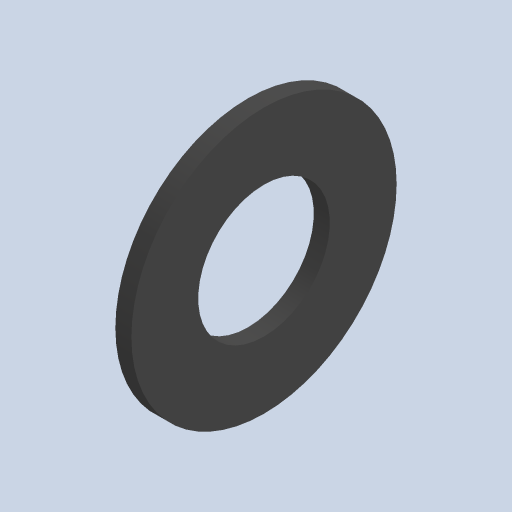
# Autodesk Inventor part: rubberWasher1
Saved by Autodesk Inventor 2023 (Build 270158030, 158C)
## iProperties
Created: 2023-01-21
Part Number: rubberWasher1
Material: Rubber
Document SubType Name: Modeling
Designer: kumpu
Density: 0.93 g/cm^3
Appearance: Rubber - Black
Author: kumpu
Autodesk Inventor part; units mm, degrees
ref_plane "YZ Plane" through (0, 0, 0) normal (1, 0, 0) x (0, 1, 0)
ref_plane "XZ Plane" through (0, 0, 0) normal (0, 1, 0) x (-1, 0, 0)
ref_plane "XY Plane" through (0, 0, 0) normal (0, 0, 1) x (1, 0, 0)
sketch "Sketch1" plane through (0, 0, 0) normal (1, 0, 0) x (0, 1, 0)
  circle A0 centre (0, 0) radius 8
  circle A1 centre (0, 0) radius 3.9688
  dimension "d0" = 16
  dimension "d1" = 7.9375
  constraints: 2 centre point, 2 coincident
  measures "d0" diameter of A0
  measures "d1" diameter of A1
extrude "Extrusion1" add sketch "Sketch1" along normal mid plane 0.9652
body "Solid1"
